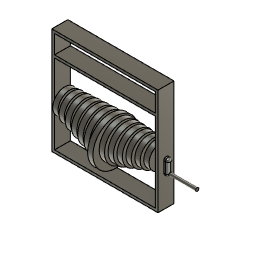
Final Project - Water Drop Mechanism v8 (Autodesk Fusion 360 design; units mm, degrees)
Autodesk Fusion 360 part; units mm, degrees
sketch "frame" plane through (0, 0, 0) normal (0, 1, 0) x (1, 0, 0) in component "frame"
  line L0 (-117.2472, -100.3536) -> (82.7528, -100.3536)
  line L1 (82.7528, -100.3536) -> (82.7528, 99.6464)
  line L2 (82.7528, 99.6464) -> (-117.2472, 99.6464)
  line L3 (-117.2472, 99.6464) -> (-117.2472, -100.3536)
  line L4 (-112.2472, -95.3536) -> (77.7528, -95.3536)
  line L5 (77.7528, 94.6464) -> (-112.2472, 94.6464)
  line L6 (-85.455, -55.3536) -> (77.7528, -55.3536)
  line L7 (-85.455, -55.3536) -> (-112.2472, -55.3536)
  line L8 (77.7528, -55.3536) -> (-112.2472, -55.3536)
  line L9 (-112.2472, -60.3536) -> (77.7528, -60.3536)
  line L10 (77.7528, -95.3536) -> (77.7528, -60.3536)
  line L11 (77.7528, -55.3536) -> (77.7528, 94.6464)
  line L12 (-112.2472, 94.6464) -> (-112.2472, -55.3536)
  line L13 (-112.2472, -60.3536) -> (-112.2472, -95.3536)
  dimension "d1" = 200
  dimension "d2" = 200
  dimension "d5" = 5
  constraint horizontal L0
  constraint vertical L1
  constraint horizontal L2
  constraint vertical L3
  constraint coincident L6.end L10
  constraint perpendicular L6 L10
  constraint perpendicular L7 L12
  constraint horizontal L8
  constraint horizontal L9
  constraint parallel L3 L12
  constraint parallel L0 L4
  constraint parallel L1 L10
  constraint parallel L2 L5
  constraint collinear L10 L11
  constraint collinear L12 L13
  measures "d1" distance of L0.start L0.end
  measures "d2" distance of L0.start L2.end
  measures "d5" distance of L6.end L9.end
extrude "Extrude1" add sketch "frame" along normal mid plane 30 makes body 1 in component "frame"
sketch "handle" plane through (82.7528, 0, 0) normal (1, 0, 0) x (0, 1, 0) in component "handle"
  line L0 (-15, -99.6464) -> (15, -99.6464)
  line L1 (15, -99.6464) -> (15, 100.3536)
  line L2 (15, 100.3536) -> (-15, 100.3536)
  line L3 (-15, 100.3536) -> (-15, -99.6464)
  line L4 (0, 55.35) -> (0, -94.6465)
  circle A0 centre (0, -19.6482) radius 4
  line L5 (-5, -19.6482) -> (-5, -39.6482)
  arc A1 (-5, -39.6482) -> (5, -39.6482) centre (0, -39.6482) ccw
  line L6 (5, -39.6482) -> (5, -19.6482)
  arc A2 (5, -19.6482) -> (-5, -19.6482) centre (0, -19.6482) ccw
  line L7 (0, -19.6482) -> (0, -39.6482) construction
  circle A3 centre (0, -39.6482) radius 3
  circle A4 centre (0, -19.6482) radius 2.53
  dimension "d8" = 8
  dimension "d9" = 20
  dimension "d10" = 6
  dimension "d39" = -1.47
  constraint perpendicular L0 L4
  constraint midpoint L4 A0.centre
  constraint tangent L5 A1
  constraint tangent A1 L6
  constraint parallel L5 L6
  constraint tangent L6 A2
  constraint tangent L5 A2
  constraint coincident L4 A1.centre
  constraint parallel L4 L7
  constraint coincident A0.centre A2.centre
  constraint concentric A1 A3
  measures "d8" diameter of A0
  measures "d9" distance of A0.centre A1.centre
  measures "d10" diameter of A3
extrude "Extrude1'" add sketch "handle" along normal blind 9 and the other way blind -1 separate body contours L4 A0 A1 L6 A2 A3 | L4 A0 L5 A1 A2 A3 | L4 A0 A4 | L4 A0 A4 | L4 A4 | L4 A4 | L4 A3 | L4 A3 makes body 2 in component "handle"
fillet "Fillet1" radius 5 1 faces at (91.7528, 1.6667, -26.3149) on bodies 2 in component "handle"
extrude "Extrude2" add sketch "handle" along normal blind 59 and the other way blind -1 contours L4 A3 | L4 A3 bodies 2 in component "handle"
extrude "Extrude2'" cut sketch "handle" against normal blind 20 contours L4 A0 A4 | L4 A0 A4 | L4 A4 | L4 A4 bodies 1 in component "frame"
sketch "axe-handle " plane through (77.7528, 0, 0) normal (-1, 0, 0) x (0, -1, 0) in component "axe"
  circle A0 centre (0, -19.6482) radius 4
  line L0 (15, 55.3536) -> (-15, 55.3536)
  line L1 (-15, 55.3536) -> (-15, -94.6464)
  line L2 (-15, -94.6464) -> (15, -94.6464)
  line L3 (15, -94.6464) -> (15, 55.3536)
  circle A1 centre (0, -19.6482) radius 2.5
  line L4 (0, -16) -> (0, -23.2855) construction
  line L5 (0, -19.6482) -> (1, -19.6482)
  line L6 (1, -19.6482) -> (1, -16.1482)
  line L7 (1, -16.1482) -> (0, -16.1482)
  line L8 (0, -16.1482) -> (0, -19.6482)
  line L9 (-1, -19.6482) -> (-1, -16.1482)
  line L10 (-1, -16.1482) -> (0, -16.1482)
  line L11 (0, -19.6482) -> (-1, -19.6482)
  line L12 (1, -19.6482) -> (1, -23.1482)
  line L13 (1, -23.1482) -> (0, -23.1482)
  line L14 (-1, -23.1482) -> (0, -23.1482)
  line L15 (-1, -19.6482) -> (-1, -23.1482)
  dimension "d22" = 5
  dimension "d23" = 5
  dimension "d24" = 1
  dimension "d25" = 3.5
  constraint concentric A0 A1
  constraint vertical L4
  constraint horizontal L5
  constraint vertical L6
  constraint horizontal L7
  constraint vertical L8
  constraint coincident A0.centre A1.centre
  constraint symmetric L4 L5.end L9.start
  constraint symmetric L4 L6.end L9.end
  constraint symmetric L4 L7.end L8.start
  constraint symmetric L6.start L5 L12.start
  constraint symmetric L6.end L5 L12.end
  constraint symmetric L7.end L5 L13.end
  constraint symmetric L5 L9.start L11.end
  constraint symmetric L5 L9.end L14.start
  constraint symmetric L5 L7.end L13.end
  measures "d22" diameter of A1
  measures "d23" diameter of A1
  measures "d24" distance of A0.centre L5.end
  measures "d25" distance of A0.centre L7.end
extrude "Extrude1''" add sketch "axe-handle " along normal blind 197 separate body contours A1 L6 L12 | A1 L5 L6 L8 | A1 L5 L11 L12 L15 | A1 L8 L9 L11 | A1 L9 L15 makes body 3 in component "axe"
sketch "axe hole" plane through (-119.2472, 0, 0) normal (-1, 0, 0) x (0, -1, 0) in component "frame"
  circle A0 centre (0, -19.6482) radius 2.5
  circle A1 centre (0, -19.6482) radius 2.8
  dimension "d28" = 0.3
extrude "Extrude3" cut sketch "axe hole" against normal blind 9 contours A0 | A1 bodies 1 in component "frame"
extrude "Extrude2''" cut sketch "axe hole" against normal blind 9 contours A0 | A1 bodies 3 in component "axe"
extrude "Extrude3'" add 1 faces at (-110.2472, -0.5244, -21.085) along direction (-1, 0, 0) blind 9 on bodies 3 bodies 3 in component "axe"
sketch "axe-end" plane through (-119.2472, 0, 0) normal (-1, 0, 0) x (0, -1, 0) in component "axe"
  circle A0 centre (0, -19.6482) radius 2.5
  circle A1 centre (0, -19.6482) radius 4.9922
  dimension "d35" = 2.4922
extrude "Extrude4" add sketch "axe-end" against normal blind 1.97 bodies 3 in component "axe"
fillet "Fillet1'" radius 4.5 1 edges at (-119.2472, 4.6544, -21.4535) on bodies 3 in component "axe"
extrude "Extrude3''" add sketch "axe-handle " against normal blind 8 contours A0 bodies 2 in component "handle"
move_face "OffsetFaces1" offset -0.02 10 faces at (79.7528, 1, -22.3424) (81.7528, 2.4971, -19.5275) (79.7528, 1, -16.9541) (79.7528, 0.6667, -23.1482) (79.7528, -0.6667, -23.1482) (81.7528, -2.1553, -18.3815) (81.7528, -2.4274, -20.2462) (79.7528, -1, -16.9541) (79.7528, -0.6667, -16.1482) (79.7528, 0.6667, -16.1482) on bodies 2 in component "handle"
extrude "Extrude5" add sketch "axe-handle " against normal blind 5.95 contours A1 L6 L12 | A1 L5 L6 L8 | A1 L6 L7 L8 | A1 L12 L13 L14 L15 | A1 L5 L11 L12 L15 | A1 L8 L9 L11 | A1 L8 L9 L10 | A1 L9 L15 bodies 3 in component "axe"
move_face "OffsetFaces2" offset -0.02 1 faces at (79.7528, 3.9244, -20.4223) on bodies 2 in component "handle"
sketch "front-view disks" plane through (0, 0, 0) normal (0, 1, 0) x (1, 0, 0)
  line L0 (-106, -2) -> (-96, -2)
  line L1 (-96, -2) -> (-96, 43)
  line L2 (-96, 43) -> (-106, 43)
  line L3 (-106, 43) -> (-106, -2)
  line L4 (-92.1827, -2) -> (-82.1827, -2)
  line L5 (-82.1827, -2) -> (-82.1827, 48)
  line L6 (-82.1827, 48) -> (-92.1827, 48)
  line L7 (-92.1827, 48) -> (-92.1827, -2)
  line L8 (-77.0431, -2) -> (-67.0431, -2)
  line L9 (-67.0431, -2) -> (-67.0431, 53)
  line L10 (-67.0431, 53) -> (-77.0431, 53)
  line L11 (-77.0431, 53) -> (-77.0431, -2)
  line L12 (-63.5626, -2) -> (-53.5626, -2)
  line L13 (-53.5626, -2) -> (-53.5626, 58)
  line L14 (-53.5626, 58) -> (-63.5626, 58)
  line L15 (-63.5626, 58) -> (-63.5626, -2)
  line L16 (-49.6674, -2) -> (-39.6674, -2)
  line L17 (-39.6674, -2) -> (-39.6674, 63)
  line L18 (-39.6674, 63) -> (-49.6674, 63)
  line L19 (-49.6674, 63) -> (-49.6674, -2)
  line L20 (-35.9795, -2) -> (-25.9795, -2)
  line L21 (-25.9795, -2) -> (-25.9795, 68)
  line L22 (-25.9795, 68) -> (-35.9795, 68)
  line L23 (-35.9795, 68) -> (-35.9795, -2)
  line L24 (-22.3668, -2) -> (-12.3668, -2)
  line L25 (-12.3668, -2) -> (-12.3668, 83)
  line L26 (-12.3668, 83) -> (-22.3668, 83)
  line L27 (-22.3668, 83) -> (-22.3668, -2)
  line L28 (-112.3602, -65.0806) -> (77.6265, -65.0806) construction
  line L29 (77.6265, -65.0806) -> (77.6265, -55.35)
  line L30 (77.6265, -55.35) -> (-112.3602, -55.35)
  line L31 (-112.3602, -55.35) -> (-112.3602, -65.0806)
  line L32 (-17.3668, -65.0806) -> (-17.3668, 61.0805) construction
  line L33 (1.2458, -2) -> (-8.7542, -2)
  line L34 (-8.7542, -2) -> (-8.7542, 68)
  line L35 (-8.7542, 68) -> (1.2458, 68)
  line L36 (1.2458, 68) -> (1.2458, -2)
  line L37 (4.9337, -2) -> (4.9337, 63)
  line L38 (4.9337, 63) -> (14.9337, 63)
  line L39 (14.9337, 63) -> (14.9337, -2)
  line L40 (14.9337, -2) -> (4.9337, -2)
  line L41 (28.829, -2) -> (18.829, -2)
  line L42 (28.829, 58) -> (28.829, -2)
  line L43 (18.829, -2) -> (18.829, 58)
  line L44 (18.829, 58) -> (28.829, 58)
  line L45 (32.3094, 53) -> (42.3094, 53)
  line L46 (42.3094, 53) -> (42.3094, -2)
  line L47 (32.3094, -2) -> (32.3094, 53)
  line L48 (42.3094, -2) -> (32.3094, -2)
  line L49 (47.4491, -2) -> (47.4491, 48)
  line L50 (57.4491, -2) -> (47.4491, -2)
  line L51 (57.4491, 48) -> (57.4491, -2)
  line L52 (47.4491, 48) -> (57.4491, 48)
  line L53 (61.2663, 43) -> (71.2663, 43)
  line L54 (71.2663, 43) -> (71.2663, -2)
  line L55 (61.2663, -2) -> (61.2663, 43)
  line L56 (71.2663, -2) -> (61.2663, -2)
  dimension "d46" = 10
  dimension "d47" = 45
  dimension "d48" = 10
  dimension "d49" = 50
  dimension "d50" = 10
  dimension "d51" = 55
  dimension "d52" = 10
  dimension "d53" = 60
  dimension "d54" = 10
  dimension "d55" = 65
  dimension "d56" = 10
  dimension "d57" = 70
  dimension "d58" = 10
  dimension "d59" = 85
  constraint horizontal L0
  constraint vertical L1
  constraint horizontal L2
  constraint vertical L3
  constraint horizontal L4
  constraint vertical L5
  constraint horizontal L6
  constraint vertical L7
  constraint horizontal L8
  constraint vertical L9
  constraint horizontal L10
  constraint vertical L11
  constraint horizontal L12
  constraint vertical L13
  constraint horizontal L14
  constraint vertical L15
  constraint horizontal L16
  constraint vertical L17
  constraint horizontal L18
  constraint vertical L19
  constraint horizontal L20
  constraint vertical L21
  constraint horizontal L22
  constraint vertical L23
  constraint horizontal L24
  constraint vertical L25
  constraint horizontal L26
  constraint vertical L27
  constraint horizontal L28
  constraint vertical L29
  constraint horizontal L30
  constraint vertical L31
  constraint midpoint L28 L32.start
  constraint perpendicular L26 L32
  constraint midpoint L24 L32
  constraint symmetric L0.start L32 L54.end
  constraint symmetric L0.end L32 L55.start
  constraint symmetric L1.end L32 L53.start
  constraint symmetric L2.end L32 L53.end
  constraint symmetric L4.start L32 L50.start
  constraint symmetric L4.end L32 L49.start
  constraint symmetric L5.end L32 L49.end
  constraint symmetric L6.end L32 L51.start
  constraint symmetric L8.start L32 L46.end
  constraint symmetric L8.end L32 L47.start
  constraint symmetric L9.end L32 L45.start
  constraint symmetric L10.end L32 L45.end
  constraint symmetric L12.start L32 L41.start
  constraint symmetric L12.end L32 L41.end
  constraint symmetric L13.end L32 L43.end
  constraint symmetric L14.end L32 L42.start
  constraint symmetric L16.start L32 L39.end
  constraint symmetric L16.end L32 L37.start
  constraint symmetric L17.end L32 L37.end
  constraint symmetric L18.end L32 L38.end
  constraint symmetric L20.start L32 L33.start
  constraint symmetric L20.end L32 L33.end
  constraint symmetric L21.end L32 L34.end
  constraint symmetric L22.end L32 L35.end
  measures "d46" distance of L0.start L0.end
  measures "d47" distance of L0.start L2.end
  measures "d48" distance of L4.start L4.end
  measures "d49" distance of L4.start L6.end
  measures "d50" distance of L8.start L8.end
  measures "d51" distance of L8.start L10.end
  measures "d52" distance of L12.start L12.end
  measures "d53" distance of L12.start L14.end
  measures "d54" distance of L16.start L16.end
  measures "d55" distance of L16.start L18.end
  measures "d56" distance of L20.start L20.end
  measures "d57" distance of L20.start L22.end
  measures "d58" distance of L24.start L24.end
  measures "d59" distance of L24.start L26.end
ref_plane "WorkPlane3" through (-106.0002, 0, -19.6464) normal (1, 0, 0) x (0, 0, -1) in component "disks"
ref_plane "WorkPlane7" through (71.5058, 0, -19.6464) normal (-1, 0, 0) x (0, 0, 1) in component "disks"
sketch "disk-45" plane through (-106.0002, 0, -19.6464) normal (1, 0, 0) x (0, 1, 0) in component "disks"
  circle A0 centre (0, 0) radius 22.5
  dimension "d67" = 45
  constraint coincident A0.centre origin
  measures "d67" diameter of A0
extrude "Extrude1'''" add sketch "disk-45" along normal blind 10 separate body makes body 4 in component "disks"
sketch "disk-45-stanga" plane through (71.5058, 0, -19.6464) normal (-1, 0, 0) x (0, 1, 0) in component "disks"
  circle A0 centre (0, 0) radius 22.5
  dimension "d70" = 45
  constraint coincident A0.centre origin
  measures "d70" diameter of A0
extrude "Extrude2'''" add sketch "disk-45-stanga" along normal blind 10 separate body makes body 5 in component "disks"
ref_plane "WorkPlane8" through (-17.2472, 0, -19.6464) normal (-1, 0, 0) x (0, 0, 1) in component "disks"
sketch "disk-85" plane through (-17.2472, 0, -19.6464) normal (-1, 0, 0) x (0, 1, 0) in component "disks"
  circle A0 centre (0, 0) radius 22.5 construction
  line L0 (0, 0) -> (0, 20)
  circle A1 centre (0, 20) radius 42.5
  dimension "d74" = 45
  dimension "d76" = 20
  dimension "d77" = 85
  constraint coincident A0.centre L0.start
  constraint vertical L0
  constraint coincident L0.end A1.centre
  measures "d74" diameter of A0
  measures "d76" distance of A0.centre L0.end
  measures "d77" diameter of A1
extrude "Extrude3'''" add sketch "disk-85" along normal mid plane 10 separate body makes body 6 in component "disks"
ref_plane "WorkPlane9" through (-7.955, 0, -39.6464) normal (1, 0, 0) x (0, -1, 0) in component "disks"
sketch "disk-70-dreapta" plane through (-7.955, 0, -39.6464) normal (1, 0, 0) x (0, 1, 0) in component "disks"
  circle A0 centre (0, 7.5) radius 35
  circle A1 centre (0, 0) radius 42.5
  dimension "d81" = 70
  constraint tangent A0 A1
  measures "d81" diameter of A0
extrude "Extrude4'" add sketch "disk-70-dreapta" along normal blind 10 separate body contours A0 makes body 7 in component "disks"
ref_plane "WorkPlane10" through (6.3372, 0, -32.1464) normal (1, 0, 0) x (0, 1, 0) in component "disks"
sketch "disk-65-dreapta" plane through (6.3372, 0, -34.6464) normal (1, 0, 0) x (0, 1, 0) in component "disks"
  circle A0 centre (0, 5) radius 32.5
  circle A1 centre (0, -5) radius 42.5
  dimension "d85" = 65
  constraint tangent A0 A1
  measures "d85" diameter of A0
extrude "Extrude5'" add sketch "disk-65-dreapta" along normal blind 10 separate body contours A0 makes body 8 in component "disks"
ref_plane "WorkPlane11" through (20.6293, 0, -29.6464) normal (1, 0, 0) x (0, 1, 0) in component "disks"
sketch "disk-60-dreapta" plane through (20.6293, 0, -32.1464) normal (1, 0, 0) x (0, 1, 0) in component "disks"
  circle A0 centre (0, 5) radius 30
  circle A1 centre (0, -7.5) radius 42.5
  dimension "d89" = 60
  constraint tangent A0 A1
  measures "d89" diameter of A0
extrude "Extrude6" add sketch "disk-60-dreapta" along normal blind 10 separate body contours A0 makes body 9 in component "disks"
ref_plane "WorkPlane12" through (34.9215, 0, -27.1464) normal (1, 0, 0) x (0, 1, 0) in component "disks"
sketch "disk-55-dreapta" plane through (34.9215, 0, -29.6464) normal (1, 0, 0) x (0, 1, 0) in component "disks"
  circle A0 centre (0, 5) radius 27.5
  circle A1 centre (0, -10) radius 42.5
  dimension "d93" = 55
  constraint tangent A0 A1
  measures "d93" diameter of A0
extrude "Extrude7" add sketch "disk-55-dreapta" along normal blind 10 separate body contours A0 makes body 10 in component "disks"
ref_plane "WorkPlane13" through (49.2137, 0, -24.6464) normal (1, 0, 0) x (0, 1, 0) in component "disks"
sketch "disk-50-dreapta" plane through (49.2137, 0, -27.1464) normal (1, 0, 0) x (0, 1, 0) in component "disks"
  circle A0 centre (0, 5) radius 25
  circle A1 centre (0, -12.5) radius 42.5
  dimension "d119" = 50
  constraint tangent A0 A1
  measures "d119" diameter of A0
extrude "Extrude8" add sketch "disk-50-dreapta" along normal blind 10 separate body contours A0 makes body 11 in component "disks"
move_body "Align1" bodies 5 to x (1, 0, 0) y (0, 1, 0) z (0, 0, 1) at (-2.2922, 0, 0) in component "disks"
move_body "Move1" bodies 5 to x (1, 0, 0) y (0, 1, 0) z (0, 0, 1) at (4.2922, 0, 0) in component "disks"
ref_plane "WorkPlane14" through (-26.5393, 0, -39.6464) normal (-1, 0, 0) x (0, 1, 0) in component "disks"
sketch "disk-70-stanga" plane through (-26.5393, 0, -39.6464) normal (-1, 0, 0) x (0, 1, 0) in component "disks"
  circle A0 centre (0, -7.5) radius 35
  circle A1 centre (0, 0) radius 42.5
  dimension "d100" = 70
  constraint tangent A0 A1
  measures "d100" diameter of A0
extrude "Extrude9" add sketch "disk-70-stanga" along normal blind 10 separate body contours A0 makes body 12 in component "disks"
ref_plane "WorkPlane15" through (-40.8315, 0, -32.1464) normal (-1, 0, 0) x (0, 1, 0) in component "disks"
sketch "disk-65-stanga" plane through (-40.8315, 0, -34.6464) normal (-1, 0, 0) x (0, 1, 0) in component "disks"
  circle A0 centre (0, -5) radius 32.5
  circle A1 centre (0, 5) radius 42.5
  dimension "d104" = 65
  constraint tangent A0 A1
  measures "d104" diameter of A0
extrude "Extrude10" add sketch "disk-65-stanga" along normal blind 10 separate body contours A0 makes body 13 in component "disks"
ref_plane "WorkPlane16" through (-55.1237, 0, -29.6464) normal (-1, 0, 0) x (0, 1, 0) in component "disks"
sketch "disk-60-stanga" plane through (-55.1237, 0, -32.1464) normal (-1, 0, 0) x (0, 1, 0) in component "disks"
  circle A0 centre (0, -5) radius 30
  circle A1 centre (0, 7.5) radius 42.5
  dimension "d108" = 60
  constraint tangent A0 A1
  measures "d108" diameter of A0
extrude "Extrude11" add sketch "disk-60-stanga" along normal blind 10 separate body contours A0 makes body 14 in component "disks"
ref_plane "WorkPlane17" through (-69.4158, 0, -27.1464) normal (-1, 0, 0) x (0, 1, 0) in component "disks"
sketch "disk-55-stanga" plane through (-69.4158, 0, -29.6464) normal (-1, 0, 0) x (0, 1, 0) in component "disks"
  circle A0 centre (0, -5) radius 27.5
  circle A1 centre (0, 10) radius 42.5
  dimension "d112" = 55
  constraint tangent A0 A1
  measures "d112" diameter of A0
extrude "Extrude12" add sketch "disk-55-stanga" along normal blind 10 separate body contours A0 makes body 15 in component "disks"
ref_plane "WorkPlane18" through (-83.708, 0, -24.6464) normal (-1, 0, 0) x (0, 1, 0) in component "disks"
sketch "disk-50-stanga" plane through (-83.708, 0, -27.1464) normal (-1, 0, 0) x (0, 1, 0) in component "disks"
  circle A0 centre (0, -5) radius 25
  dimension "d116" = 50
  measures "d116" diameter of A0
extrude "Extrude13" add sketch "disk-50-stanga" along normal blind 10 separate body makes body 16 in component "disks"
move_body "Align2" bodies 4 to x (1, 0, 0) y (0, 1, 0) z (0, 0, 1) at (2.2922, 0, 0) in component "disks"
move_body "Move2" bodies 4 to x (1, 0, 0) y (0, 1, 0) z (0, 0, 1) at (-4.2922, 0, 0) in component "disks"
sketch "axe hole (2)" plane through (73.5058, 0, 0) normal (1, 0, 0) x (0, 1, 0) in component "disks"
  circle A0 centre (0, -19.6464) radius 22.5
  circle A1 centre (0, -19.6464) radius 2.65
  dimension "d120" = 5.3
  constraint concentric A0 A1
  measures "d120" diameter of A1
extrude "Extrude14" cut sketch "axe hole (2)" against normal blind 190 contours A1 bodies 4 5 6 7 8 9 10 11 12 13 14 15 16 in component "disks"
ref_plane "WorkPlane1" through (-17.2472, 0, -19.6464) normal (-1, 0, 0) x (0, 0, 1)
component "frame" placed x (1, 0, 0) y (0, 1, 0) z (0, 0, 1) at (0, 0, 0)
component "handle" placed x (1, 0, 0) y (0, 1, 0) z (0, 0, 1) at (0, 0, 0)
component "disks" placed x (1, 0, 0) y (0, 1, 0) z (0, 0, 1) at (0, 0, 0)
component "axe" placed x (1, 0, 0) y (0, 1, 0) z (0, 0, 1) at (0, 0, 0)
component "circles" placed x (1, 0, 0) y (0, 1, 0) z (0, 0, 1) at (0, 0, 0)
equation "d76 = ( 85 / 2 ) * 1 mm - ( 45 / 2 ) * 1 mm"
equation "d80 = ( 25.753 / 6 ) * 1 mm"
equation "d84 = ( 25.753 / 6 ) * 1 mm"
equation "d88 = ( 25.753 / 6 ) * 1 mm"
equation "d92 = ( 25.753 / 6 ) * 1 mm"
equation "d96 = ( 25.753 / 6 ) * 1 mm"
equation "d99 = ( 25.753 / 6 ) * 1 mm"
equation "d103 = ( 25.753 / 6 ) * 1 mm"
equation "d107 = ( 25.753 / 6 ) * 1 mm"
equation "d111 = ( 25.753 / 6 ) * 1 mm"
equation "d115 = ( 25.753 / 6 ) * 1 mm"
named bodies: "frame", "handle", "45-left", "45-right", "85", "70-right", "65-right", "60-right", "55-right", "50-right", "70-left", "65-left", "60-left", "55-left", "50-left"
